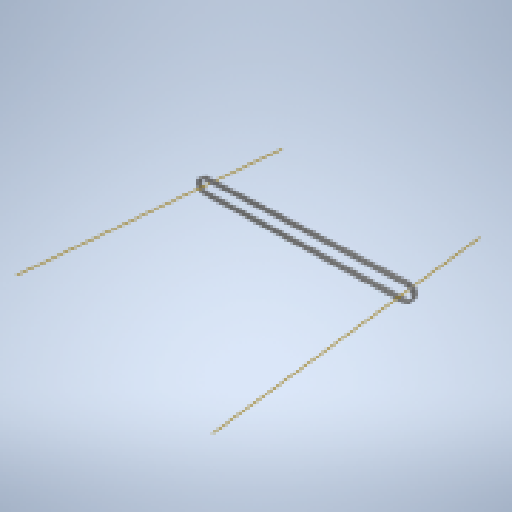
# Autodesk Inventor part: Synchronous Belt
Saved by Autodesk Inventor 2023 (Build 270158000, 158)
## iProperties
Created: 2022-10-18
Part Number: Synchronous Belt
Material: Rubber
Document SubType Name: Modeling
Designer: klebe
Density: 1 g/cm^3
Appearance: Rubber - Black - Version 1.1
CustomPartVersion: 1
Author: klebe
Autodesk Inventor part; units mm, degrees
sketch "Sketch Path" plane through (0, 0, 0) normal (0, 0, 1) x (1, 0, 0)
  arc A0 (0.0029, 5.4577) -> (-0.0012, -10.4577) centre (0.0008, -2.5) ccw
  arc A1 (219.8695, -10.5144) -> (219.8736, 5.4011) centre (219.8716, -2.5566) ccw
  line L0 (219.8695, -10.5144) -> (-0.0012, -10.4577)
  line L1 (0.0029, 5.4577) -> (219.8736, 5.4011)
  constraints: 4 end point, 4 point on circle, 2 centre point
ref_plane "Cross Section Plane" through (-0.0012, -10.4577, 0) normal (1, -0.0003, 0) x (0, 0, 1)
ref_plane "Work Plane2" through (0.0008, -2.5, 0) normal (-1, 0, 0) x (0, 0, 1)
ref_plane "Work Plane3" through (219.8716, -2.5566, 0) normal (-0.9999, 0.0162, 0) x (0, 0, 1)
sketch "Cross Section" plane through (-0.0012, -10.4577, 0) normal (1, -0.0003, 0) x (0, 0, 1)
  line L0 (-3, 0.5) -> (3, 0.5)
  line L1 (3, 0.5) -> (3, -0.5)
  line L2 (3, -0.5) -> (-3, -0.5)
  line L3 (-3, -0.5) -> (-3, 0.5)
  line L4 (-3, 0) -> (3, 0) construction
  point P0 (0, 0)
  point P1 (0, 0)
  dimension "d0" = 6
  dimension "d4" = 0.5
  dimension "d5" = 0.5
  constraints: 10 end point, 3 midpoint, 2 parallel, 1 coincident, 1 horizontal, 1 perpendicular, 1 other
  measures "d0" distance between parallel lines of L1 L3
  measures "d4" distance between parallel lines of L2 L4
  measures "d5" distance between parallel lines of L4 L0
sweep "Belt" add profiles "Cross Section" path "Sketch Path"
equation "\"d0\" = da_B"
equation "\"d4\" = da_a"
equation "\"d5\" = da_a2"
equation "\"da_B\" = 6"
equation "\"da_pb\" = 5"
equation "\"da_L\" = 489.74157"
equation "\"da_a\" = 0.5"
equation "\"da_S\" = 2.65"
equation "\"da_Beta\" = 20deg"
equation "\"da_Ht\" = 1.2"
equation "\"da_H\" = 2.2"
equation "\"da_a2\" = 0.5"
body "Solid1"
